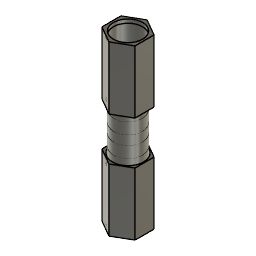
Microbot Case (Autodesk Fusion 360 design; units mm, degrees)
Autodesk Fusion 360 part; units mm, degrees
sketch "Sketch1" plane through (0, 0, 0) normal (0, 0, 1) x (1, 0, 0) in component "PCB"
  circle A0 centre (0, 0) radius 7.75
  dimension "d1" = 15.5
  constraint coincident A0.centre origin
  measures "d1" diameter of A0
extrude "Extrude1" add sketch "Sketch1" along normal blind 6.2 makes body 1 in component "PCB"
move_body "Move1" bodies 1 to x (1, 0, 0) y (0, 1, 0) z (0, 0, 1) at (0, 0, 2.5) in component "PCB"
mirror "Mirror1" about plane through (0, 0, 0) normal (0, 0, 1) of bodies 1 makes body 2 in component "PCB"
sketch "Sketch2" plane through (0, 0, 2.5) normal (0, 0, -1) x (1, 0, 0) in component "Central Case"
  circle A0 centre (0, 0) radius 7.75
  circle A1 centre (0, 0) radius 7.9
  circle A2 centre (0, 0) radius 8.1
  dimension "d7" = 15.8
  dimension "d8" = 16.2
  constraint coincident A0.centre A1.centre
  measures "d7" diameter of A1
  measures "d8" diameter of A2
extrude "Extrude1'" add sketch "Sketch2" along normal blind 2.5 separate body contours A2 makes body 3 in component "Central Case"
extrude "Extrude2" add sketch "Sketch2" against normal blind 6.25 contours A2 bodies 3 in component "Central Case"
extrude "Extrude3" add 1 faces at (-7.529, 2.7435, 8.75) along direction (0, 0, 1) blind 5 on bodies 3 bodies 3 in component "Central Case"
extrude "Extrude1''" add sketch "Sketch2" against normal blind 3 from surface at -11.25 separate body contours A0 | A1 makes body 4
fillet "Fillet1" radius 7.5 1 faces at (0.3823, -1.6751, 16.75) on bodies 4
extrude "Extrude2'" cut 1 faces at (-0.423, 0.3925, 16.75) along direction (0, 0, -1) blind 3 on bodies 4 bodies 4
mirror "Mirror1'" about plane through (0, 0, 0) normal (0, 0, 1) of bodies 4 makes body 5
mirror "Mirror1''" about plane through (0, 0, 0) normal (0, 0, 1) of bodies 3 merged in component "Central Case"
sketch "Sketch1 (2)" plane through (0, 0, 13.75) normal (0, 0, -1) x (1, 0, 0) in component "Arm"
  circle A0 centre (0, 0) radius 1.9
  circle A1 centre (0, 0) radius 7.9
  circle A2 centre (0, 0) radius 8.5
  line L0 (9, 5.1962) -> (0, 10.3923)
  line L1 (0, 10.3923) -> (-9, 5.1962)
  line L2 (-9, 5.1962) -> (-9, -5.1962)
  line L3 (-9, -5.1962) -> (0, -10.3923)
  line L4 (0, -10.3923) -> (9, -5.1962)
  line L5 (9, -5.1962) -> (9, 5.1962)
  constraint coincident A0.centre A1.centre
extrude "Extrude1'''" add sketch "Sketch1 (2)" along normal blind 2 separate body contours L0 L1 L2 L3 L4 L5 makes body 6 in component "Arm"
extrude "Extrude2''" add 1 faces at (-7.8938, 4.5575, 13.75) along direction (0, 0, 1) blind 2 on bodies 6 bodies 6 in component "Arm"
extrude "Extrude3'" add sketch "Sketch1 (2)" against normal blind 1 from surface at -1 contours A2 bodies 6 in component "Arm"
extrude "Extrude4" add sketch "Sketch1 (2)" against normal blind 30 from surface at -2 contours L0 L1 L2 L3 L4 L5 bodies 6 in component "Arm"
extrude "Extrude5" add sketch "Sketch1 (2)" against normal blind 2 from surface at -30 contours A2 | L0 L1 L2 L3 L4 L5 bodies 6 in component "Arm"
mirror "Mirror1'''" about plane through (0, 0, 0) normal (0, 0, 1) of bodies 6 makes body 7 in component "Arm"
component "PCB" placed x (1, 0, 0) y (0, 1, 0) z (0, 0, 1) at (0, 0, 0)
component "Central Case" placed x (1, 0, 0) y (0, 1, 0) z (0, 0, 1) at (0, 0, 0)
component "Arm" placed x (1, 0, 0) y (0, 1, 0) z (0, 0, 1) at (0, 0, 0)
